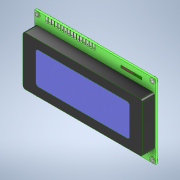
# Autodesk Inventor part: Part1_Pantalla_LCD_20x4
Saved by Autodesk Inventor 2021 (Build 250183000, 183)
## iProperties
Created: 2022-06-25
Part Number: Part1_Pantalla_LCD_20x4
Material: Generic
Document SubType Name: Modeling
Designer: Sam14
Density: 1 g/cm^3
Appearance: Chrome - Polished
Author: Sam14
Autodesk Inventor part; units mm, degrees
ref_plane "YZ Plane" through (0, 0, 0) normal (1, 0, 0) x (0, 1, 0)
ref_plane "XZ Plane" through (0, 0, 0) normal (0, 1, 0) x (-1, 0, 0)
ref_plane "XY Plane" through (0, 0, 0) normal (0, 0, 1) x (1, 0, 0)
sketch "Sketch1" plane through (0, 0, 0) normal (0, 0, 1) x (1, 0, 0)
  line L0 (48.95, -30) -> (-48.95, -30)
  line L1 (-48.95, -30) -> (-48.95, 30)
  line L2 (-48.95, 30) -> (48.95, 30)
  line L3 (48.95, 30) -> (48.95, -30)
  line L4 (48.95, -30) -> (-48.95, 30) construction
  line L5 (-48.95, -30) -> (48.95, 30) construction
  circle A0 centre (-46.7, -27.75) radius 1.65
  circle A1 centre (-46.7, 27.75) radius 1.65
  circle A2 centre (46.7, 27.75) radius 1.65
  circle A3 centre (46.7, -27.75) radius 1.65
  line L6 (-48.95, 30) -> (-38.95, 30)
  line L7 (-38.95, 30) -> (-38.95, 27)
  line L8 (-38.95, 30) -> (-39.95, 30)
  line L9 (-38.95, 30) -> (-37.95, 30)
  line L10 (-38.63, 26.68) -> (-39.27, 26.68)
  line L11 (-39.27, 26.68) -> (-39.27, 27.32)
  line L12 (-39.27, 27.32) -> (-38.63, 27.32)
  line L13 (-38.63, 27.32) -> (-38.63, 26.68)
  line L14 (-38.63, 26.68) -> (-39.27, 27.32) construction
  line L15 (-39.27, 26.68) -> (-38.63, 27.32) construction
  line L16 (-36.09, 26.68) -> (-36.73, 26.68)
  line L17 (-36.73, 26.68) -> (-36.73, 27.32)
  line L18 (-36.73, 27.32) -> (-36.09, 27.32)
  line L19 (-36.09, 27.32) -> (-36.09, 26.68)
  line L20 (-33.55, 26.68) -> (-34.19, 26.68)
  line L21 (-34.19, 26.68) -> (-34.19, 27.32)
  line L22 (-34.19, 27.32) -> (-33.55, 27.32)
  line L23 (-33.55, 27.32) -> (-33.55, 26.68)
  line L24 (-31.01, 26.68) -> (-31.65, 26.68)
  line L25 (-31.65, 26.68) -> (-31.65, 27.32)
  line L26 (-31.65, 27.32) -> (-31.01, 27.32)
  line L27 (-31.01, 27.32) -> (-31.01, 26.68)
  line L28 (-28.47, 26.68) -> (-29.11, 26.68)
  line L29 (-29.11, 26.68) -> (-29.11, 27.32)
  line L30 (-29.11, 27.32) -> (-28.47, 27.32)
  line L31 (-28.47, 27.32) -> (-28.47, 26.68)
  line L32 (-25.93, 26.68) -> (-26.57, 26.68)
  line L33 (-26.57, 26.68) -> (-26.57, 27.32)
  line L34 (-26.57, 27.32) -> (-25.93, 27.32)
  line L35 (-25.93, 27.32) -> (-25.93, 26.68)
  line L36 (-23.39, 26.68) -> (-24.03, 26.68)
  line L37 (-24.03, 26.68) -> (-24.03, 27.32)
  line L38 (-24.03, 27.32) -> (-23.39, 27.32)
  line L39 (-23.39, 27.32) -> (-23.39, 26.68)
  line L40 (-20.85, 26.68) -> (-21.49, 26.68)
  line L41 (-21.49, 26.68) -> (-21.49, 27.32)
  line L42 (-21.49, 27.32) -> (-20.85, 27.32)
  line L43 (-20.85, 27.32) -> (-20.85, 26.68)
  line L44 (-18.31, 26.68) -> (-18.95, 26.68)
  line L45 (-18.95, 26.68) -> (-18.95, 27.32)
  line L46 (-18.95, 27.32) -> (-18.31, 27.32)
  line L47 (-18.31, 27.32) -> (-18.31, 26.68)
  line L48 (-15.77, 26.68) -> (-16.41, 26.68)
  line L49 (-16.41, 26.68) -> (-16.41, 27.32)
  line L50 (-16.41, 27.32) -> (-15.77, 27.32)
  line L51 (-15.77, 27.32) -> (-15.77, 26.68)
  line L52 (-13.23, 26.68) -> (-13.87, 26.68)
  line L53 (-13.87, 26.68) -> (-13.87, 27.32)
  line L54 (-13.87, 27.32) -> (-13.23, 27.32)
  line L55 (-13.23, 27.32) -> (-13.23, 26.68)
  line L56 (-10.69, 26.68) -> (-11.33, 26.68)
  line L57 (-11.33, 26.68) -> (-11.33, 27.32)
  line L58 (-11.33, 27.32) -> (-10.69, 27.32)
  line L59 (-10.69, 27.32) -> (-10.69, 26.68)
  line L60 (-8.15, 26.68) -> (-8.79, 26.68)
  line L61 (-8.79, 26.68) -> (-8.79, 27.32)
  line L62 (-8.79, 27.32) -> (-8.15, 27.32)
  line L63 (-8.15, 27.32) -> (-8.15, 26.68)
  line L64 (-5.61, 26.68) -> (-6.25, 26.68)
  line L65 (-6.25, 26.68) -> (-6.25, 27.32)
  line L66 (-6.25, 27.32) -> (-5.61, 27.32)
  line L67 (-5.61, 27.32) -> (-5.61, 26.68)
  line L68 (-3.07, 26.68) -> (-3.71, 26.68)
  line L69 (-3.71, 26.68) -> (-3.71, 27.32)
  line L70 (-3.71, 27.32) -> (-3.07, 27.32)
  line L71 (-3.07, 27.32) -> (-3.07, 26.68)
  line L72 (-0.53, 26.68) -> (-1.17, 26.68)
  line L73 (-1.17, 26.68) -> (-1.17, 27.32)
  line L74 (-1.17, 27.32) -> (-0.53, 27.32)
  line L75 (-0.53, 27.32) -> (-0.53, 26.68)
  point P0 (0, 0)
  dimension "d0" = 97.9
  dimension "d1" = 60
  dimension "d3" = 3.3
  dimension "d4" = 3.3
  dimension "d5" = 3.3
  dimension "d6" = 3.3
  dimension "d11" = 10
  dimension "d12" = 3
  dimension "d15" = 1
  dimension "d16" = 1
  dimension "d17" = 0.64
  dimension "d18" = 0.64
  dimension "d20" = 0.64
  dimension "d21" = 0.64
  dimension "d23" = 0.64
  dimension "d24" = 0.64
  dimension "d26" = 0.64
  dimension "d27" = 0.64
  dimension "d29" = 0.64
  dimension "d30" = 0.64
  dimension "d32" = 0.64
  dimension "d33" = 0.64
  dimension "d35" = 0.64
  dimension "d36" = 0.64
  dimension "d38" = 0.64
  dimension "d39" = 0.64
  dimension "d41" = 0.64
  dimension "d42" = 0.64
  dimension "d44" = 0.64
  dimension "d45" = 0.64
  dimension "d47" = 0.64
  dimension "d48" = 0.64
  dimension "d50" = 0.64
  dimension "d51" = 0.64
  dimension "d53" = 0.64
  dimension "d54" = 0.64
  dimension "d56" = 0.64
  dimension "d57" = 0.64
  dimension "d59" = 0.64
  dimension "d60" = 0.64
  dimension "d62" = 0.64
  dimension "d63" = 0.64
  constraints: 152 end point, 34 parallel, 18 perpendicular, 4 centre point, 3 point on line, 2 midpoint, 1 horizontal, 1 vertical
  measures "d0" distance of L0.start L0.end
  measures "d1" distance of L0.end L1.end
  measures "d3" diameter of A0
  measures "d4" diameter of A1
  measures "d5" diameter of A2
  measures "d6" diameter of A3
  measures "d11" distance of L1.end L6.end
  measures "d12" distance of L6.end L7.end
  measures "d15" distance of L6.end L8.end
  measures "d16" distance of L6.end L9.end
  measures "d17" distance of L10.start L10.end
  measures "d18" distance of L10.end L11.end
  measures "d20" distance of L19.end L16.end
  measures "d21" distance of L16.end L17.end
  measures "d23" distance of L23.end L20.end
  measures "d24" distance of L20.end L21.end
  measures "d26" distance of L27.end L24.end
  measures "d27" distance of L24.end L25.end
  measures "d29" distance of L31.end L28.end
  measures "d30" distance of L28.end L29.end
  measures "d32" distance of L35.end L32.end
  measures "d33" distance of L32.end L33.end
  measures "d35" distance of L39.end L36.end
  measures "d36" distance of L36.end L37.end
  measures "d38" distance of L43.end L40.end
  measures "d39" distance of L40.end L41.end
  measures "d41" distance of L47.end L44.end
  measures "d42" distance of L44.end L45.end
  measures "d44" distance of L51.end L48.end
  measures "d45" distance of L48.end L49.end
  measures "d47" distance of L55.end L52.end
  measures "d48" distance of L52.end L53.end
  measures "d50" distance of L59.end L56.end
  measures "d51" distance of L56.end L57.end
  measures "d53" distance of L63.end L60.end
  measures "d54" distance of L60.end L61.end
  measures "d56" distance of L67.end L64.end
  measures "d57" distance of L64.end L65.end
  measures "d59" distance of L71.end L68.end
  measures "d60" distance of L68.end L69.end
  measures "d62" distance of L75.end L72.end
  measures "d63" distance of L72.end L73.end
extrude "Extrusion1" add sketch "Sketch1" along normal blind 1.5
sketch "Sketch4" plane through (0, 0, 1.5) normal (0, 0, 1) x (1, 0, 0)
  line L0 (-48.95, 30) -> (-48.95, -30) projected
  line L1 (-48.95, -30) -> (48.95, -30) projected
  line L2 (48.95, -30) -> (48.95, 30) projected
  line L3 (48.95, 30) -> (-48.95, 30) projected
  line L4 (-39.27, 27.32) -> (-38.63, 27.32) projected
  line L5 (-38.63, 27.32) -> (-38.63, 26.68) projected
  line L6 (-38.63, 26.68) -> (-39.27, 26.68) projected
  line L7 (-39.27, 26.68) -> (-39.27, 27.32) projected
  circle A0 centre (-46.7, -27.75) radius 1.65 projected
  circle A1 centre (-46.7, 27.75) radius 1.65 projected
  circle A2 centre (46.7, 27.75) radius 1.65 projected
  circle A3 centre (46.7, -27.75) radius 1.65 projected
  line L8 (-0.53, 27.32) -> (-0.53, 26.68) projected
  line L9 (-0.53, 26.68) -> (-1.17, 26.68) projected
  line L10 (-1.17, 26.68) -> (-1.17, 27.32) projected
  line L11 (-1.17, 27.32) -> (-0.53, 27.32) projected
  line L12 (-3.07, 27.32) -> (-3.07, 26.68) projected
  line L13 (-3.07, 26.68) -> (-3.71, 26.68) projected
  line L14 (-3.71, 26.68) -> (-3.71, 27.32) projected
  line L15 (-3.71, 27.32) -> (-3.07, 27.32) projected
  line L16 (-5.61, 27.32) -> (-5.61, 26.68) projected
  line L17 (-5.61, 26.68) -> (-6.25, 26.68) projected
  line L18 (-6.25, 26.68) -> (-6.25, 27.32) projected
  line L19 (-6.25, 27.32) -> (-5.61, 27.32) projected
  line L20 (-8.15, 27.32) -> (-8.15, 26.68) projected
  line L21 (-8.15, 26.68) -> (-8.79, 26.68) projected
  line L22 (-8.79, 26.68) -> (-8.79, 27.32) projected
  line L23 (-8.79, 27.32) -> (-8.15, 27.32) projected
  line L24 (-10.69, 27.32) -> (-10.69, 26.68) projected
  line L25 (-10.69, 26.68) -> (-11.33, 26.68) projected
  line L26 (-11.33, 26.68) -> (-11.33, 27.32) projected
  line L27 (-11.33, 27.32) -> (-10.69, 27.32) projected
  line L28 (-13.23, 27.32) -> (-13.23, 26.68) projected
  line L29 (-13.23, 26.68) -> (-13.87, 26.68) projected
  line L30 (-13.87, 26.68) -> (-13.87, 27.32) projected
  line L31 (-13.87, 27.32) -> (-13.23, 27.32) projected
  line L32 (-15.77, 27.32) -> (-15.77, 26.68) projected
  line L33 (-15.77, 26.68) -> (-16.41, 26.68) projected
  line L34 (-16.41, 26.68) -> (-16.41, 27.32) projected
  line L35 (-16.41, 27.32) -> (-15.77, 27.32) projected
  line L36 (-18.31, 27.32) -> (-18.31, 26.68) projected
  line L37 (-18.31, 26.68) -> (-18.95, 26.68) projected
  line L38 (-18.95, 26.68) -> (-18.95, 27.32) projected
  line L39 (-18.95, 27.32) -> (-18.31, 27.32) projected
  line L40 (-20.85, 27.32) -> (-20.85, 26.68) projected
  line L41 (-20.85, 26.68) -> (-21.49, 26.68) projected
  line L42 (-21.49, 26.68) -> (-21.49, 27.32) projected
  line L43 (-21.49, 27.32) -> (-20.85, 27.32) projected
  line L44 (-23.39, 27.32) -> (-23.39, 26.68) projected
  line L45 (-23.39, 26.68) -> (-24.03, 26.68) projected
  line L46 (-24.03, 26.68) -> (-24.03, 27.32) projected
  line L47 (-24.03, 27.32) -> (-23.39, 27.32) projected
  line L48 (-25.93, 27.32) -> (-25.93, 26.68) projected
  line L49 (-25.93, 26.68) -> (-26.57, 26.68) projected
  line L50 (-26.57, 26.68) -> (-26.57, 27.32) projected
  line L51 (-26.57, 27.32) -> (-25.93, 27.32) projected
  line L52 (-28.47, 27.32) -> (-28.47, 26.68) projected
  line L53 (-28.47, 26.68) -> (-29.11, 26.68) projected
  line L54 (-29.11, 26.68) -> (-29.11, 27.32) projected
  line L55 (-29.11, 27.32) -> (-28.47, 27.32) projected
  line L56 (-31.01, 27.32) -> (-31.01, 26.68) projected
  line L57 (-31.01, 26.68) -> (-31.65, 26.68) projected
  line L58 (-31.65, 26.68) -> (-31.65, 27.32) projected
  line L59 (-31.65, 27.32) -> (-31.01, 27.32) projected
  line L60 (-33.55, 27.32) -> (-33.55, 26.68) projected
  line L61 (-33.55, 26.68) -> (-34.19, 26.68) projected
  line L62 (-34.19, 26.68) -> (-34.19, 27.32) projected
  line L63 (-34.19, 27.32) -> (-33.55, 27.32) projected
  line L64 (-36.09, 27.32) -> (-36.09, 26.68) projected
  line L65 (-36.09, 26.68) -> (-36.73, 26.68) projected
  line L66 (-36.73, 26.68) -> (-36.73, 27.32) projected
  line L67 (-36.73, 27.32) -> (-36.09, 27.32) projected
  circle A4 centre (-46.7, 27.75) radius 2.25
  circle A5 centre (-46.7, -27.75) radius 2.25
  circle A6 centre (46.7, -27.75) radius 2.25
  circle A7 centre (46.7, 27.75) radius 2.25
  line L68 (-38.95, 30) -> (-37.95, 30)
  line L69 (48.95, 30) -> (-48.95, 30) projected
  line L70 (-37.95, 30) -> (-37.95, 26)
  line L71 (-38.95, 30) -> (-39.95, 30)
  line L72 (-39.95, 30) -> (-39.95, 26)
  line L73 (-38.95, 25.5) -> (-39.95, 26)
  line L74 (-39.95, 26) -> (-38.95, 25.5)
  line L75 (-37.95, 26) -> (-38.95, 25.5)
  line L76 (-36.41, 30) -> (-35.41, 30)
  line L77 (-35.41, 30) -> (-35.41, 26)
  line L78 (-36.41, 30) -> (-37.41, 30)
  line L79 (-37.41, 30) -> (-37.41, 26)
  line L80 (-37.41, 26) -> (-36.41, 25.5)
  line L81 (-35.41, 26) -> (-36.41, 25.5)
  line L82 (-33.87, 30) -> (-32.87, 30)
  line L83 (-32.87, 30) -> (-32.87, 26)
  line L84 (-33.87, 30) -> (-34.87, 30)
  line L85 (-34.87, 30) -> (-34.87, 26)
  line L86 (-34.87, 26) -> (-33.87, 25.5)
  line L87 (-32.87, 26) -> (-33.87, 25.5)
  line L88 (-31.33, 30) -> (-30.33, 30)
  line L89 (-30.33, 30) -> (-30.33, 26)
  line L90 (-31.33, 30) -> (-32.33, 30)
  line L91 (-32.33, 30) -> (-32.33, 26)
  line L92 (-32.33, 26) -> (-31.33, 25.5)
  line L93 (-30.33, 26) -> (-31.33, 25.5)
  line L94 (-28.79, 30) -> (-27.79, 30)
  line L95 (-27.79, 30) -> (-27.79, 26)
  line L96 (-28.79, 30) -> (-29.79, 30)
  line L97 (-29.79, 30) -> (-29.79, 26)
  line L98 (-29.79, 26) -> (-28.79, 25.5)
  line L99 (-27.79, 26) -> (-28.79, 25.5)
  line L100 (-26.25, 30) -> (-25.25, 30)
  line L101 (-25.25, 30) -> (-25.25, 26)
  line L102 (-26.25, 30) -> (-27.25, 30)
  line L103 (-27.25, 30) -> (-27.25, 26)
  line L104 (-27.25, 26) -> (-26.25, 25.5)
  line L105 (-25.25, 26) -> (-26.25, 25.5)
  line L106 (-23.71, 30) -> (-22.71, 30)
  line L107 (-22.71, 30) -> (-22.71, 26)
  line L108 (-23.71, 30) -> (-24.71, 30)
  line L109 (-24.71, 30) -> (-24.71, 26)
  line L110 (-24.71, 26) -> (-23.71, 25.5)
  line L111 (-22.71, 26) -> (-23.71, 25.5)
  line L112 (-21.17, 30) -> (-20.17, 30)
  line L113 (-20.17, 30) -> (-20.17, 26)
  line L114 (-21.17, 30) -> (-22.17, 30)
  line L115 (-22.17, 30) -> (-22.17, 26)
  line L116 (-22.17, 26) -> (-21.17, 25.5)
  line L117 (-20.17, 26) -> (-21.17, 25.5)
  line L118 (-18.63, 30) -> (-17.63, 30)
  line L119 (-17.63, 30) -> (-17.63, 26)
  line L120 (-18.63, 30) -> (-19.63, 30)
  line L121 (-19.63, 30) -> (-19.63, 26)
  line L122 (-19.63, 26) -> (-18.63, 25.5)
  line L123 (-17.63, 26) -> (-18.63, 25.5)
  line L124 (-16.09, 30) -> (-15.09, 30)
  line L125 (-15.09, 30) -> (-15.09, 26)
  line L126 (-16.09, 30) -> (-17.09, 30)
  line L127 (-17.09, 30) -> (-17.09, 26)
  line L128 (-17.09, 26) -> (-16.09, 25.5)
  line L129 (-15.09, 26) -> (-16.09, 25.5)
  line L130 (-13.55, 30) -> (-12.55, 30)
  line L131 (-12.55, 30) -> (-12.55, 26)
  line L132 (-13.55, 30) -> (-14.55, 30)
  line L133 (-14.55, 30) -> (-14.55, 26)
  line L134 (-14.55, 26) -> (-13.55, 25.5)
  line L135 (-12.55, 26) -> (-13.55, 25.5)
  line L136 (-11.01, 30) -> (-10.01, 30)
  line L137 (-10.01, 30) -> (-10.01, 26)
  line L138 (-11.01, 30) -> (-12.01, 30)
  line L139 (-12.01, 30) -> (-12.01, 26)
  line L140 (-12.01, 26) -> (-11.01, 25.5)
  line L141 (-10.01, 26) -> (-11.01, 25.5)
  line L142 (-8.47, 30) -> (-7.47, 30)
  line L143 (-7.47, 30) -> (-7.47, 26)
  line L144 (-8.47, 30) -> (-9.47, 30)
  line L145 (-9.47, 30) -> (-9.47, 26)
  line L146 (-9.47, 26) -> (-8.47, 25.5)
  line L147 (-7.47, 26) -> (-8.47, 25.5)
  line L148 (-5.93, 30) -> (-4.93, 30)
  line L149 (-4.93, 30) -> (-4.93, 26)
  line L150 (-5.93, 30) -> (-6.93, 30)
  line L151 (-6.93, 30) -> (-6.93, 26)
  line L152 (-6.93, 26) -> (-5.93, 25.5)
  line L153 (-4.93, 26) -> (-5.93, 25.5)
  line L154 (-3.39, 30) -> (-2.39, 30)
  line L155 (-2.39, 30) -> (-2.39, 26)
  line L156 (-3.39, 30) -> (-4.39, 30)
  line L157 (-4.39, 30) -> (-4.39, 26)
  line L158 (-4.39, 26) -> (-3.39, 25.5)
  line L159 (-2.39, 26) -> (-3.39, 25.5)
  line L160 (-0.85, 30) -> (0.15, 30)
  line L161 (0.15, 30) -> (0.15, 26)
  line L162 (-0.85, 30) -> (-1.85, 30)
  line L163 (-1.85, 30) -> (-1.85, 26)
  line L164 (-1.85, 26) -> (-0.85, 25.5)
  line L165 (0.15, 26) -> (-0.85, 25.5)
  point P0 (0, 0)
  dimension "d64" = 1
  dimension "d65" = 1
  dimension "d67" = 1
  dimension "d68" = 1
  dimension "d69" = 1
  dimension "d70" = 1
  dimension "d71" = 1
  dimension "d72" = 1
  dimension "d73" = 1
  dimension "d74" = 1
  dimension "d75" = 1
  dimension "d76" = 1
  dimension "d77" = 1
  dimension "d78" = 1
  dimension "d79" = 1
  dimension "d80" = 1
  dimension "d81" = 1
  dimension "d82" = 1
  dimension "d83" = 1
  dimension "d84" = 1
  dimension "d85" = 1
  dimension "d86" = 1
  dimension "d87" = 1
  dimension "d88" = 1
  dimension "d89" = 1
  dimension "d90" = 1
  dimension "d91" = 1
  dimension "d92" = 1
  dimension "d93" = 1
  dimension "d94" = 1
  dimension "d95" = 1
  dimension "d96" = 1
  constraints: 194 end point, 16 perpendicular, 4 centre point, 2 point on line, 1 coincident, 1 collinear, 1 vertical, 3 other
  measures "d64" distance of L68.start L68.end
  measures "d65" distance of L68.start L71.end
  measures "d67" distance of L78.start L77.start
  measures "d68" distance of L78.start L78.end
  measures "d69" distance of L84.start L83.start
  measures "d70" distance of L84.start L84.end
  measures "d71" distance of L90.start L89.start
  measures "d72" distance of L90.start L90.end
  measures "d73" distance of L96.start L95.start
  measures "d74" distance of L96.start L96.end
  measures "d75" distance of L102.start L101.start
  measures "d76" distance of L102.start L102.end
  measures "d77" distance of L108.start L107.start
  measures "d78" distance of L108.start L108.end
  measures "d79" distance of L114.start L113.start
  measures "d80" distance of L114.start L114.end
  measures "d81" distance of L120.start L119.start
  measures "d82" distance of L120.start L120.end
  measures "d83" distance of L126.start L125.start
  measures "d84" distance of L126.start L126.end
  measures "d85" distance of L132.start L131.start
  measures "d86" distance of L132.start L132.end
  measures "d87" distance of L138.start L137.start
  measures "d88" distance of L138.start L138.end
  measures "d89" distance of L144.start L143.start
  measures "d90" distance of L144.start L144.end
  measures "d91" distance of L150.start L149.start
  measures "d92" distance of L150.start L150.end
  measures "d93" distance of L156.start L155.start
  measures "d94" distance of L156.start L156.end
  measures "d95" distance of L162.start L161.start
  measures "d96" distance of L162.start L162.end
extrude "Extrusion3" add sketch "Sketch4" along normal blind 0.25 and the other way blind 1.75 contours A4 | A5 | L3 L70 L75 L73 L72 | A6 | L3 L77 L81 L80 L79 | A7 | L161 L165 L164 L163 L3 | L3 L83 L87 L86 L85 | L155 L159 L158 L157 L3 | L3 L89 L93 L92 L91 | L149 L153 L152 L151 L3 | L3 L95 L99 L98 L97 | L143 L147 L146 L145 L3 | L3 L101 L105 L104 L103 | L137 L141 L140 L139 L3 | L3 L107 L111 L110 L109 | L131 L135 L134 L133 L3 | L3 L113 L117 L116 L115 | L125 L129 L128 L127 L3 | L3 L119 L123 L122 L121
sketch "Sketch5" plane through (0, 0, 1.5) normal (0, 0, 1) x (1, 0, 0)
  line L0 (46.5, 20) -> (-46.5, 20)
  line L1 (-48.5, 18) -> (-48.5, -18)
  line L2 (-46.5, -20) -> (46.5, -20)
  line L3 (48.5, -18) -> (48.5, 18)
  line L4 (48.5, 20) -> (-48.5, -20) construction
  line L5 (-48.5, 20) -> (48.5, -20) construction
  arc A0 (-46.5, 20) -> (-48.5, 18) centre (-46.5, 18) ccw
  arc A1 (48.5, 18) -> (46.5, 20) centre (46.5, 18) ccw
  arc A2 (46.5, -20) -> (48.5, -18) centre (46.5, -18) ccw
  arc A3 (-48.5, -18) -> (-46.5, -20) centre (-46.5, -18) ccw
  point P0 (0, 0)
  dimension "d101" = 97
  dimension "d102" = 40
  dimension "d103" = 2
  constraints: 12 end point, 8 point on circle, 8 point on line, 8 tangent, 4 centre point, 3 equal radius, 2 midpoint, 2 parallel, 1 horizontal, 1 perpendicular
  measures "d101" distance of L4.start L5.start
  measures "d102" distance of L4.end L5.start
  measures "d103" radius of A0
extrude "Extrusion4" add sketch "Sketch5" along normal blind 10
sketch "Sketch6" plane through (0, 0, 11.5) normal (0, 0, 1) x (1, 0, 0)
  line L0 (36, -13) -> (-36, -13)
  line L1 (-38, -11) -> (-38, 11)
  line L2 (-36, 13) -> (36, 13)
  line L3 (38, 11) -> (38, -11)
  line L4 (38, -13) -> (-38, 13) construction
  line L5 (-38, -13) -> (38, 13) construction
  arc A0 (-36, 13) -> (-38, 11) centre (-36, 11) ccw
  arc A1 (38, 11) -> (36, 13) centre (36, 11) ccw
  arc A2 (36, -13) -> (38, -11) centre (36, -11) ccw
  arc A3 (-38, -11) -> (-36, -13) centre (-36, -11) ccw
  point P0 (0, 0)
  dimension "d106" = 76
  dimension "d107" = 26
  dimension "d108" = 2
  constraints: 12 end point, 8 point on circle, 8 point on line, 8 tangent, 4 centre point, 3 equal radius, 2 midpoint, 2 parallel, 1 horizontal, 1 perpendicular
  measures "d106" distance of L4.start L5.start
  measures "d107" distance of L5.start L4.end
  measures "d108" radius of A0
extrude "Extrusion5" cut sketch "Sketch6" against normal blind 5
sketch "Sketch9" plane through (0, 0, 11.5) normal (0, 0, 1) x (1, 0, 0)
  line L0 (-36, 13) -> (36, 13) projected
  arc A0 (-36, 13) -> (-38, 11) centre (-36, 11) ccw projected
  line L1 (-38, -11) -> (-38, 11) projected
  arc A1 (-38, -11) -> (-36, -13) centre (-36, -11) ccw projected
  line L2 (36, -13) -> (-36, -13) projected
  arc A2 (36, -13) -> (38, -11) centre (36, -11) ccw projected
  line L3 (38, 11) -> (38, -11) projected
  arc A3 (38, 11) -> (36, 13) centre (36, 11) ccw projected
  point P0 (0, 0)
extrude "Extrusion7" add sketch "Sketch9" against normal blind 1 separate body
sketch "Sketch10" plane through (0, 0, 1.5) normal (0, 0, 1) x (1, 0, 0)
  line L0 (20.95, 26) -> (37.95, 26)
  line L1 (37.95, 26) -> (37.95, 23.9)
  line L2 (37.95, 23.9) -> (20.95, 23.9)
  line L3 (20.95, 23.9) -> (20.95, 26)
  point P0 (0, 0)
  point P1 (48.95, 30)
  dimension "d117" = 17
  dimension "d118" = 2.1
  constraints: 8 end point, 3 perpendicular
  measures "d117" distance of L0.start L0.end
  measures "d118" distance of L0.end L1.end
extrude "Extrusion8" cut sketch "Sketch10" against normal blind 0.2 bodies 1
sketch "Sketch11" plane through (0, 0, 1.3) normal (0, 0, 1) x (1, 0, 0)
  line L0 (30.0122, 25.8896) -> (41.0024, 25.8896) construction
  line L1 (41.0024, 25.8896) -> (41.0024, 20.1599) construction
  line L2 (41.0024, 20.1599) -> (30.0122, 20.1599) construction
  line L3 (30.0122, 20.1599) -> (30.0122, 25.8896) construction
  line L4 (31.3225, 23.9496) -> (30.1508, 23.9496)
  line L5 (30.1508, 23.9496) -> (30.1508, 24.219)
  spline S0 degree 2 poles (30.1508, 24.219) (30.277, 24.3376) (30.5018, 24.5577) (30.6096, 24.6763) knots 0 0 0 1 2 2 2
  spline S1 degree 2 poles (30.6096, 24.6763) (30.8267, 24.915) (30.9853, 25.2013) (30.9853, 25.3538) knots 0 0 0 1 2 2 2
  spline S2 degree 2 poles (30.9853, 25.3538) (30.9853, 25.4338) (30.936, 25.5539) (30.8914, 25.5924) knots 0 0 0 1 2 2 2
  spline S3 degree 2 poles (30.8914, 25.5924) (30.8467, 25.6309) (30.7297, 25.6694) (30.6589, 25.6694) knots 0 0 0 1 2 2 2
  spline S4 degree 2 poles (30.6589, 25.6694) (30.5911, 25.6694) (30.4526, 25.6355) (30.3894, 25.6094) knots 0 0 0 1 2 2 2
  spline S5 degree 2 poles (30.3894, 25.6094) (30.3355, 25.5878) (30.2355, 25.5262) (30.2047, 25.5047) knots 0 0 0 1 2 2 2
  line L6 (30.2047, 25.5047) -> (30.1908, 25.5047)
  line L7 (30.1908, 25.5047) -> (30.1908, 25.7757)
  spline S6 degree 2 poles (30.1908, 25.7757) (30.2693, 25.8141) (30.5511, 25.8896) (30.6773, 25.8896) knots 0 0 0 1 2 2 2
  spline S7 degree 2 poles (30.6773, 25.8896) (30.9437, 25.8896) (31.244, 25.6078) (31.244, 25.3676) knots 0 0 0 1 2 2 2
  spline S8 degree 2 poles (31.244, 25.3676) (31.244, 25.2552) (31.1916, 25.0674) (31.1454, 24.9873) knots 0 0 0 1 2 2 2
  spline S9 degree 2 poles (31.1454, 24.9873) (31.0992, 24.9042) (30.9653, 24.741) (30.8914, 24.6624) knots 0 0 0 1 2 2 2
  spline S10 degree 2 poles (30.8914, 24.6624) (30.7713, 24.5316) (30.4772, 24.2513) (30.3894, 24.1697) knots 0 0 0 1 2 2 2
  line L8 (30.3894, 24.1697) -> (31.3225, 24.1697)
  line L9 (31.3225, 24.1697) -> (31.3225, 23.9496)
  spline S11 degree 2 poles (32.759, 24.8996) (32.759, 24.3884) (32.4619, 23.9095) (32.1524, 23.9095) knots 0 0 0 1 2 2 2
  spline S12 degree 2 poles (32.1524, 23.9095) (31.8383, 23.9095) (31.5442, 24.3976) (31.5442, 24.898) knots 0 0 0 1 2 2 2
  spline S13 degree 2 poles (31.5442, 24.898) (31.5442, 25.4123) (31.8414, 25.8881) (32.1524, 25.8881) knots 0 0 0 1 2 2 2
  spline S14 degree 2 poles (32.1524, 25.8881) (32.4649, 25.8881) (32.759, 25.3953) (32.759, 24.8996) knots 0 0 0 1 2 2 2
  spline S15 degree 2 poles (32.4326, 24.3206) (32.4696, 24.4145) (32.5004, 24.704) (32.5004, 24.8996) knots 0 0 0 1 2 2 2
  spline S16 degree 2 poles (32.5004, 24.8996) (32.5004, 25.0951) (32.4696, 25.383) (32.4311, 25.48) knots 0 0 0 1 2 2 2
  spline S17 degree 2 poles (32.4311, 25.48) (32.3926, 25.577) (32.2586, 25.6771) (32.1524, 25.6771) knots 0 0 0 1 2 2 2
  spline S18 degree 2 poles (32.1524, 25.6771) (32.0461, 25.6771) (31.9091, 25.577) (31.8691, 25.4769) knots 0 0 0 1 2 2 2
  spline S19 degree 2 poles (31.8691, 25.4769) (31.8306, 25.3799) (31.8029, 25.0843) (31.8029, 24.898) knots 0 0 0 1 2 2 2
  spline S20 degree 2 poles (31.8029, 24.898) (31.8029, 24.6979) (31.8275, 24.4299) (31.8675, 24.3252) knots 0 0 0 1 2 2 2
  spline S21 degree 2 poles (31.8675, 24.3252) (31.9045, 24.2267) (32.0415, 24.1205) (32.1524, 24.1205) knots 0 0 0 1 2 2 2
  spline S22 degree 2 poles (32.1524, 24.1205) (32.2571, 24.1205) (32.3941, 24.2205) (32.4326, 24.3206) knots 0 0 0 1 2 2 2
  spline S23 degree 2 poles (34.1848, 24.8996) (34.1848, 24.3884) (33.8876, 23.9095) (33.5782, 23.9095) knots 0 0 0 1 2 2 2
  spline S24 degree 2 poles (33.5782, 23.9095) (33.2641, 23.9095) (32.97, 24.3976) (32.97, 24.898) knots 0 0 0 1 2 2 2
  spline S25 degree 2 poles (32.97, 24.898) (32.97, 25.4123) (33.2671, 25.8881) (33.5782, 25.8881) knots 0 0 0 1 2 2 2
  spline S26 degree 2 poles (33.5782, 25.8881) (33.8907, 25.8881) (34.1848, 25.3953) (34.1848, 24.8996) knots 0 0 0 1 2 2 2
  spline S27 degree 2 poles (33.8584, 24.3206) (33.8953, 24.4145) (33.9261, 24.704) (33.9261, 24.8996) knots 0 0 0 1 2 2 2
  spline S28 degree 2 poles (33.9261, 24.8996) (33.9261, 25.0951) (33.8953, 25.383) (33.8568, 25.48) knots 0 0 0 1 2 2 2
  spline S29 degree 2 poles (33.8568, 25.48) (33.8184, 25.577) (33.6844, 25.6771) (33.5782, 25.6771) knots 0 0 0 1 2 2 2
  spline S30 degree 2 poles (33.5782, 25.6771) (33.4719, 25.6771) (33.3349, 25.577) (33.2949, 25.4769) knots 0 0 0 1 2 2 2
  spline S31 degree 2 poles (33.2949, 25.4769) (33.2564, 25.3799) (33.2286, 25.0843) (33.2286, 24.898) knots 0 0 0 1 2 2 2
  spline S32 degree 2 poles (33.2286, 24.898) (33.2286, 24.6979) (33.2533, 24.4299) (33.2933, 24.3252) knots 0 0 0 1 2 2 2
  spline S33 degree 2 poles (33.2933, 24.3252) (33.3303, 24.2267) (33.4673, 24.1205) (33.5782, 24.1205) knots 0 0 0 1 2 2 2
  spline S34 degree 2 poles (33.5782, 24.1205) (33.6829, 24.1205) (33.8199, 24.2205) (33.8584, 24.3206) knots 0 0 0 1 2 2 2
  line L10 (35.6506, 24.6024) -> (35.4243, 24.6024)
  line L11 (35.4243, 24.6024) -> (35.4243, 23.9496)
  line L12 (35.4243, 23.9496) -> (35.1795, 23.9496)
  line L13 (35.1795, 23.9496) -> (35.1795, 24.6024)
  line L14 (35.1795, 24.6024) -> (34.3403, 24.6024)
  line L15 (34.3403, 24.6024) -> (34.3403, 24.8703)
  line L16 (34.3403, 24.8703) -> (35.1902, 25.8496)
  line L17 (35.1902, 25.8496) -> (35.4243, 25.8496)
  line L18 (35.4243, 25.8496) -> (35.4243, 24.8072)
  line L19 (35.4243, 24.8072) -> (35.6506, 24.8072)
  line L20 (35.6506, 24.8072) -> (35.6506, 24.6024)
  line L21 (35.1795, 24.8072) -> (35.1795, 25.5493)
  line L22 (35.1795, 25.5493) -> (34.5405, 24.8072)
  line L23 (34.5405, 24.8072) -> (35.1795, 24.8072)
  line L24 (35.703, 23.9496) -> (36.3435, 25.8496)
  line L25 (36.3435, 25.8496) -> (36.6545, 25.8496)
  line L26 (36.6545, 25.8496) -> (37.295, 23.9496)
  line L27 (37.295, 23.9496) -> (37.0286, 23.9496)
  line L28 (37.0286, 23.9496) -> (36.8562, 24.4808)
  line L29 (36.8562, 24.4808) -> (36.131, 24.4808)
  line L30 (36.131, 24.4808) -> (35.9585, 23.9496)
  line L31 (35.9585, 23.9496) -> (35.703, 23.9496)
  line L32 (36.7869, 24.6963) -> (36.4928, 25.5909)
  line L33 (36.4928, 25.5909) -> (36.2003, 24.6963)
  line L34 (36.2003, 24.6963) -> (36.7869, 24.6963)
  point P0 (0, 0)
  constraints: 2 other
extrude "Extrusion9" add sketch "Sketch11" along normal blind 0.2 bodies 1
body "Solid1"
body "Solid3"
